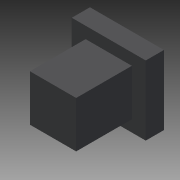
# Autodesk Inventor part: RFSplitter
Saved by Autodesk Inventor 2014 (Build 180170000, 170)
## iProperties
Created: 2015-03-25
Part Number: RFSplitter
Material: Generic
Document SubType Name: Modeling
Designer: Owner
Density: 1 g/cm^3
Appearance: Gray
Author: Owner
Autodesk Inventor part; units mm, degrees
ref_plane "YZ Plane" through (0, 0, 0) normal (1, 0, 0) x (0, 1, 0)
ref_plane "XZ Plane" through (0, 0, 0) normal (0, 1, 0) x (-1, 0, 0)
ref_plane "XY Plane" through (0, 0, 0) normal (0, 0, 1) x (1, 0, 0)
sketch "Sketch1" plane through (0, 0, 0) normal (0, 0, 1) x (1, 0, 0)
  line L0 (7.0175, -2.5627) -> (11.0815, -2.5627)
  line L1 (11.0815, -2.5627) -> (11.0815, -6.3727)
  line L2 (11.0815, -6.3727) -> (7.0175, -6.3727)
  line L3 (7.0175, -6.3727) -> (7.0175, -2.5627)
  point P0 (0, 0)
  dimension "d0" = 4.064
  dimension "d1" = 3.81
  constraints: 8 end point, 2 parallel, 1 horizontal, 1 perpendicular
  measures "d0" distance of L0.start L0.end
  measures "d1" distance of L0.end L1.end
extrude "Extrusion1" add sketch "Sketch1" along normal blind 1
sketch "Sketch2" plane through (0, 0, 1) normal (0, 0, 1) x (1, 0, 0)
  line L0 (11.0815, -2.5627) -> (7.0175, -2.5627) projected
  line L1 (11.0815, -6.3727) -> (11.0815, -2.5627) projected
  line L2 (7.7795, -3.1977) -> (10.3195, -3.1977)
  line L3 (10.3195, -3.1977) -> (10.3195, -5.7377)
  line L4 (10.3195, -5.7377) -> (7.7795, -5.7377)
  line L5 (7.7795, -5.7377) -> (7.7795, -3.1977)
  point P0 (0, 0)
  dimension "d4" = 2.54
  dimension "d5" = 2.54
  dimension "d6" = 0.635
  dimension "d7" = 0.762
  constraints: 8 end point, 2 parallel, 1 horizontal, 1 perpendicular
  measures "d4" distance of L2.start L2.end
  measures "d5" distance of L2.end L3.end
  measures "d6" distance between parallel lines of L0 L2
  measures "d7" distance between parallel lines of L1 L3
extrude "Extrusion2" add sketch "Sketch2" along normal blind 3.06
body "Solid1"
